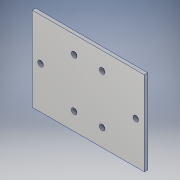
# Autodesk Inventor part: VEX Motor Mount
Saved by Autodesk Inventor 2019 (Build 230136000, 136)
## iProperties
Created: 2018-11-29
Part Number: VEX Motor Mount
Material: Aluminum 6061
Document SubType Name: Modeling
Designer: Alex Barnett
Density: 2.7 g/cm^3
Appearance: Aluminum - Flat
Author: Alex Barnett
Autodesk Inventor part; units mm, degrees
ref_plane "YZ Plane" through (0, 0, 0) normal (1, 0, 0) x (0, 1, 0)
ref_plane "XZ Plane" through (0, 0, 0) normal (0, 1, 0) x (-1, 0, 0)
ref_plane "XY Plane" through (0, 0, 0) normal (0, 0, 1) x (1, 0, 0)
sketch "Sketch1" plane through (0, 0, 0) normal (0, 0, 1) x (1, 0, 0)
  line L0 (-50.8, -38.1) -> (50.8, -38.1)
  line L1 (50.8, -38.1) -> (50.8, 38.1)
  line L2 (50.8, 38.1) -> (-50.8, 38.1)
  line L3 (-50.8, 38.1) -> (-50.8, -38.1)
  line L4 (-50.8, -38.1) -> (50.8, 38.1) construction
  line L5 (50.8, -38.1) -> (-50.8, 38.1) construction
  point P0 (0, 0)
  dimension "d0" = 101.6
  dimension "d1" = 76.2
  constraints: 12 end point, 2 midpoint, 2 parallel, 1 horizontal, 1 perpendicular
  measures "d0" distance of L2.end L1.end
  measures "d1" distance of L1.end L0.end
extrude "Extrusion1" add sketch "Sketch1" against normal blind 3.175
sketch "Sketch2" plane through (0, 0, 0) normal (0, 0, 1) x (1, 0, 0)
  circle A0 centre (43.18, 0) radius 2.54
  line L0 (50.8, -38.1) -> (50.8, 38.1) projected
  line L1 (0, 38.1) -> (0, -38.1) construction
  circle A1 centre (-43.18, 0) radius 2.54
  point P0 (0, 0)
  dimension "d4" = 5.08
  dimension "d5" = 7.62
  constraints: 2 centre point, 2 end point, 1 symmetric about line, 1 vertical, 1 other
  measures "d4" diameter of A0
  measures "d5" distance from line of L0 A0.centre
hole "Hole1" at (-43.18, 0, 0) at (43.18, 0, 0) direction (0, 0, -1) diameter 5.08 end through all
sketch "Sketch3" plane through (0, 0, 0) normal (0, 0, 1) x (1, 0, 0)
  line L0 (0, 29.2764) -> (0, -24.7835) construction
  line L1 (50.8, 38.1) -> (-50.8, 38.1) construction
  line L2 (-18.9862, 0) -> (21.3051, 0) construction
  point P0 (0, 0)
  point P1 (-12.7, 22.225)
  point P2 (0, 38.1)
  point P3 (12.7, 22.225)
  point P4 (-12.7, -22.225)
  point P5 (12.7, -22.225)
  dimension "d13" = 22.225
  dimension "d14" = 12.7
  constraints: 4 end point, 3 symmetric about line, 1 horizontal, 1 midpoint, 1 point on line, 1 vertical
  measures "d13" vertical distance of point (0, 0) point (-12.7, 22.225)
  measures "d14" distance from line of L0 point (-12.7, 22.225)
hole "Hole2" at (-12.7, 22.225, 0) at (12.7, 22.225, 0) at (-12.7, -22.225, 0) at (12.7, -22.225, 0) direction (0, 0, -1) diameter 5.08 end through all
body "Solid1"
